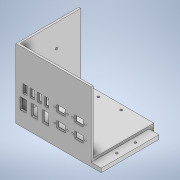
# Autodesk Inventor part: Quarter4
Saved by Autodesk Inventor 2020.2 (Build 242310000, 310)
## iProperties
Created: 2020-01-16
Part Number: Quarter4
Material: Generic
Document SubType Name: Modeling
Designer: ColinP
Density: 1 g/cm^3
Appearance: Default
Author: ColinP
Autodesk Inventor part; units mm, degrees
ref_plane "YZ Plane" through (0, 0, 0) normal (1, 0, 0) x (0, 1, 0)
ref_plane "XZ Plane" through (0, 0, 0) normal (0, 1, 0) x (-1, 0, 0)
ref_plane "XY Plane" through (0, 0, 0) normal (0, 0, 1) x (1, 0, 0)
sketch "Sketch1" plane through (0, 0, 0) normal (0, 1, 0) x (-1, 0, 0)
  line L0 (0, 0) -> (150, 0)
  line L1 (150, 0) -> (150, 125)
  line L2 (150, 125) -> (0, 125)
  line L3 (0, 125) -> (0, 0)
  dimension "d0" = 150
  dimension "d1" = 125
  constraints: 8 end point, 2 parallel, 1 horizontal, 1 perpendicular
  measures "d0" distance of L2.end L1.end
  measures "d1" distance of L1.end L0.end
extrude "Extrusion1" add sketch "Sketch1" along normal blind 10
sketch "Sketch2" plane through (0, 10, 0) normal (0, 1, 0) x (1, 0, 0)
  line L0 (0, -125) -> (0, 0) projected
  line L1 (0, 0) -> (-146, 0)
  line L2 (-146, 0) -> (-146, -121)
  line L3 (-146, -121) -> (0, -121)
  line L4 (0, -121) -> (0, 0)
  line L5 (0, -125) -> (0, 0) projected
  line L6 (0, 0) -> (-150, 0) projected
  line L7 (-150, 0) -> (-150, -125) projected
  line L8 (-150, -125) -> (0, -125) projected
  point P0 (-146, 0)
  dimension "d4" = 146
  dimension "d5" = 121
  constraints: 8 end point, 2 parallel, 1 horizontal, 1 perpendicular
  measures "d4" distance of L3.end L2.end
  measures "d5" distance of L2.end L1.end
extrude "Extrusion2" add sketch "Sketch2" along normal blind 125 contours L8 L7 L6 L2 L3 L0
sketch "Sketch3" plane through (0, 0, 125) normal (1, 0, 0) x (0, 0, -1)
  line L0 (0, 0) -> (0, 135) projected
  line L1 (0, 0) -> (0, 5)
  line L2 (125, 0) -> (125, 10) projected
  line L3 (125, 0) -> (0, 0) projected
  line L4 (125, 0) -> (0, 0)
  line L5 (0, 5) -> (115, 5)
  line L6 (115, 5) -> (125, 5)
  line L7 (115, 5) -> (115, 0)
  line L8 (0, 0) -> (125, 0) projected
  dimension "d8" = 5
  dimension "d95" = 125
  dimension "d96" = 115
  constraints: 10 end point, 2 horizontal, 2 point on line, 1 midpoint, 1 perpendicular
  measures "d8" distance of L0.start L1.end
  measures "d95" distance of L2.start L0.start
  measures "d96" distance of L1.end L5.end
sketch "Sketch4" plane through (0, 10, 121) normal (0, 0, -1) x (-1, 0, 0)
  line L0 (0, 20) -> (16, 20)
  line L1 (16, 20) -> (32.7, 20)
  line L2 (32.7, 20) -> (32.7, 32.9)
  line L3 (32.7, 32.9) -> (16, 32.9)
  line L4 (16, 32.9) -> (16, 20)
  line L5 (16, 26.45) -> (13, 26.45)
  line L6 (13, 26.45) -> (11.5, 26.45)
  circle A0 centre (11.5, 26.45) radius 1.5
  line L7 (32.7, 26.45) -> (37.2, 26.45)
  circle A1 centre (37.2, 26.45) radius 1.5
  line L8 (16, 32.9) -> (16, 47.9)
  line L9 (16, 47.9) -> (32.7, 47.9)
  line L10 (32.7, 47.9) -> (32.7, 60.8)
  line L11 (32.7, 60.8) -> (16, 60.8)
  line L12 (16, 60.8) -> (16, 47.9)
  line L13 (16, 54.35) -> (11.5, 54.35)
  line L14 (11.5, 54.35) -> (37.2, 54.35)
  circle A2 centre (11.5, 54.35) radius 1.5
  circle A3 centre (37.2, 54.35) radius 1.5
  line L15 (47.2, 54.35) -> (51.7, 54.35)
  line L16 (51.7, 54.35) -> (51.7, 47.9)
  line L17 (51.7, 47.9) -> (68.4, 47.9)
  line L18 (68.4, 47.9) -> (68.4, 60.8)
  line L19 (68.4, 60.8) -> (51.7, 60.8)
  line L20 (51.7, 60.8) -> (51.7, 54.35)
  line L21 (68.4, 54.35) -> (72.9, 54.35)
  circle A4 centre (47.2, 54.35) radius 1.5
  circle A5 centre (72.9, 54.35) radius 1.5
  line L22 (0, 0) -> (0, 125) projected
  line L23 (0, 20) -> (0, 0)
  line L24 (51.7, 32.9) -> (51.7, 20)
  line L25 (51.7, 20) -> (68.4, 20)
  line L26 (68.4, 20) -> (68.4, 32.9)
  line L27 (68.4, 32.9) -> (51.7, 32.9)
  line L28 (68.4, 26.45) -> (72.9, 26.45)
  line L29 (72.9, 26.45) -> (47.2, 26.45)
  circle A6 centre (47.2, 26.45) radius 1.5
  circle A7 centre (72.9, 26.45) radius 1.5
  line L30 (68.4, 47.9) -> (68.4, 32.9)
  line L31 (37.2, 54.35) -> (47.2, 54.35)
  point P0 (0, -10)
  dimension "d12" = 16
  dimension "d13" = 16.7
  dimension "d14" = 12.9
  dimension "d15" = 3
  dimension "d16" = 1.5
  dimension "d17" = 4.5
  dimension "d18" = 3
  dimension "d19" = 15
  dimension "d20" = 12.9
  dimension "d23" = 4.5
  dimension "d25" = 4.5
  dimension "d29" = 3
  dimension "d30" = 3
  dimension "d57" = 20
  dimension "d58" = 3
  dimension "d59" = 3
  dimension "d60" = 16.7
  dimension "d62" = 15
  dimension "d73" = 3
  dimension "d74" = 10
  dimension "d75" = 4.5
  dimension "d76" = 16.7
  dimension "d77" = 16.7
  constraints: 62 end point, 17 perpendicular, 8 coincident, 7 centre point, 7 horizontal, 6 point on line, 5 midpoint, 2 collinear, 1 horizontal alignment, 1 vertical, 2 other
  measures "d12" distance of L0.start L0.end
  measures "d13" distance of L0.end L1.end
  measures "d14" distance of L1.end L2.end
  measures "d15" distance of L5.start L5.end
  measures "d16" distance of L5.end L6.end
  measures "d17" distance of L7.start L7.end
  measures "d18" diameter of A1
  measures "d19" distance of L3.end L8.end
  measures "d20" distance of L9.end L10.end
  measures "d23" distance of L15.start L15.end
  measures "d25" distance of L21.start L21.end
  measures "d29" diameter of A4
  measures "d30" diameter of A5
  measures "d57" distance of L0.start L22.start
  measures "d58" diameter of A6
  measures "d59" diameter of A7
  measures "d60" distance of L10.end L11.end
  measures "d62" distance of L17.end L26.end
  measures "d73" diameter of A3
  measures "d74" distance of L31.start L31.end
  measures "d75" distance from line of L10 L14.end
  measures "d76" distance of L26.end L24.start
  measures "d77" distance of L16.end L17.end
extrude "Extrusion4" cut sketch "Sketch4" against normal blind 125 contours L4 L3 L2 L1 | L26 L29 L24 L27 | L20 L19 L18 L17 L16 | L12 L14 L10 L9 | L12 L11 L10 L14 | L26 L25 L24 L29
hole "Hole1" at (-11.5, 64.35, 121) at (-37.2, 64.35, 121) at (-47.2, 64.35, 121) at (-72.9, 64.35, 121) at (-37.2, 36.45, 121) at (-11.5, 36.45, 121) at (-47.2, 36.45, 121) at (-72.9, 36.45, 121) direction (0, 0, 1) diameter 3 end through all
sketch "Sketch5" plane through (-150, 135, 125) normal (0, 0, 1) x (1, 0, 0)
  circle A0 centre (77.1, -70.65) radius 1.5 projected
  line L0 (77.1, -70.65) -> (65.6, -70.65)
  line L1 (65.6, -70.65) -> (65.6, -62.3)
  line L2 (65.6, -62.3) -> (65.6, -79)
  line L3 (65.6, -79) -> (57.5, -79)
  line L4 (57.5, -79) -> (57.5, -62.3)
  line L5 (57.5, -62.3) -> (65.6, -62.3)
  line L6 (57.5, -62.3) -> (51.1, -62.3)
  line L7 (51.1, -62.3) -> (36.6, -62.3)
  line L8 (51.1, -62.3) -> (43, -62.3)
  line L9 (43, -62.3) -> (43, -79)
  line L10 (43, -79) -> (51.1, -79)
  line L11 (51.1, -79) -> (51.1, -62.3)
  line L12 (36.6, -62.3) -> (28.5, -62.3)
  line L13 (28.5, -62.3) -> (28.5, -79)
  line L14 (28.5, -79) -> (36.6, -79)
  line L15 (36.6, -79) -> (36.6, -62.3)
  line L16 (28.5, -62.3) -> (22.1, -62.3)
  line L17 (22.1, -62.3) -> (14, -62.3)
  line L18 (14, -62.3) -> (14, -79)
  line L19 (14, -79) -> (22.1, -79)
  line L20 (22.1, -79) -> (22.1, -62.3)
  point P0 (150, -135)
  point P1 (43, -62.3)
  dimension "d41" = 11.5
  dimension "d43" = 8.35
  dimension "d44" = 16.7
  dimension "d45" = 8.1
  dimension "d46" = 6.4
  dimension "d47" = 14.5
  dimension "d48" = 8.1
  dimension "d49" = 16.7
  dimension "d50" = 8.1
  dimension "d51" = 16.7
  dimension "d52" = 6.4
  dimension "d53" = 8.1
  dimension "d54" = 16.7
  constraints: 42 end point, 6 horizontal, 6 parallel, 6 perpendicular, 2 point on line, 1 vertical
  measures "d41" distance of L0.start L0.end
  measures "d43" distance of L0.end L1.end
  measures "d44" distance of L1.end L2.end
  measures "d45" distance of L2.end L3.end
  measures "d46" distance of L4.end L6.end
  measures "d47" distance of L6.end L7.end
  measures "d48" distance of L10.end L9.end
  measures "d49" distance of L9.end L8.end
  measures "d50" distance of L14.end L13.end
  measures "d51" distance of L13.end L12.end
  measures "d52" distance of L12.end L16.end
  measures "d53" distance of L19.end L18.end
  measures "d54" distance of L18.end L17.end
extrude "Extrusion5" cut sketch "Sketch5" against normal blind 10 contours L20 L19 L18 L17 | L15 L14 L13 L12 | L11 L10 L9 L7 | L2 L3 L4 L5 L1
sketch "Sketch8" plane through (-150, 135, 125) normal (0, 0, 1) x (1, 0, 0)
  circle A0 centre (77.1, -98.55) radius 1.5 projected
  line L0 (77.1, -98.55) -> (65.6, -98.55)
  line L1 (65.6, -98.55) -> (65.6, -87.25)
  line L2 (65.6, -87.25) -> (65.6, -109.85)
  line L3 (65.6, -109.85) -> (53.1, -109.85)
  line L4 (53.1, -109.85) -> (53.1, -87.25)
  line L5 (53.1, -87.25) -> (65.6, -87.25)
  line L6 (53.1, -87.25) -> (43.1, -87.25)
  line L7 (43.1, -87.25) -> (43.1, -109.85)
  line L8 (43.1, -109.85) -> (30.6, -109.85)
  line L9 (30.6, -109.85) -> (30.6, -87.25)
  line L10 (30.6, -87.25) -> (43.1, -87.25)
  line L11 (30.6, -87.25) -> (20.6, -87.25)
  line L12 (20.6, -87.25) -> (20.6, -109.85)
  line L13 (20.6, -109.85) -> (8.1, -109.85)
  line L14 (8.1, -109.85) -> (8.1, -87.25)
  line L15 (8.1, -87.25) -> (20.6, -87.25)
  dimension "d63" = 11.5
  dimension "d64" = 11.3
  dimension "d65" = 22.6
  dimension "d66" = 12.5
  dimension "d67" = 10
  dimension "d68" = 12.5
  dimension "d69" = 10
  dimension "d70" = 22.6
  dimension "d71" = 12.5
  dimension "d113" = 22.6
  constraints: 32 end point, 10 perpendicular, 6 point on line, 2 horizontal
  measures "d63" distance of L0.start L0.end
  measures "d64" distance of L0.end L1.end
  measures "d65" distance of L1.end L2.end
  measures "d66" distance of L2.end L3.end
  measures "d67" distance of L4.end L6.end
  measures "d68" distance of L7.end L8.end
  measures "d69" distance of L9.end L11.end
  measures "d70" distance of L11.end L12.end
  measures "d71" distance of L12.end L13.end
  measures "d113" distance of L13.end L14.end
extrude "Extrusion6" cut sketch "Sketch8" against normal blind 10 contours L12 L13 L14 L15 | L7 L8 L9 L10 | L2 L3 L4 L5 L1
sketch "Sketch9" plane through (-146, 10, 121) normal (1, 0, 0) x (0, 0, -1)
  line L0 (0, 0) -> (0, 125) projected
  line L1 (0, 125) -> (50, 125)
  line L2 (0, 125) -> (121, 125) projected
  line L3 (50, 125) -> (50, 85)
  line L4 (50, 85) -> (95, 85)
  line L5 (95, 85) -> (95, 28)
  line L6 (95, 28) -> (50, 28)
  line L7 (50, 28) -> (50, 85)
  line L8 (72.5, 85) -> (72.5, 80)
  line L9 (72.5, 80) -> (72.5, 33)
  circle A0 centre (72.5, 80) radius 2.5
  circle A1 centre (72.5, 33) radius 2.5
  point P0 (121, -10)
  dimension "d80" = 50
  dimension "d81" = 40
  dimension "d82" = 45
  dimension "d83" = 57
  dimension "d84" = 5
  dimension "d85" = 47
  dimension "d86" = 5
  dimension "d87" = 5
  constraints: 16 end point, 4 perpendicular, 2 centre point, 2 coincident, 2 point on line, 1 horizontal, 1 midpoint, 1 vertical
  measures "d80" distance of L0.end L1.end
  measures "d81" distance of L1.end L3.end
  measures "d82" distance of L3.end L4.end
  measures "d83" distance of L4.end L5.end
  measures "d84" distance of L8.start L8.end
  measures "d85" distance of L8.end L9.end
  measures "d86" diameter of A0
  measures "d87" diameter of A1
hole "Hole2" at (-146, 90, 48.5) at (-146, 43, 48.5) direction (-1, 0, 0) diameter 4.318 end through all
extrude "Extrusion7" add sketch "Sketch3" along normal blind 20 contours L0 L5 L7 L3
sketch "Sketch10" plane through (0, 0, 0) normal (0, -1, 0) x (1, 0, 0)
  point P0 (0, 0)
sketch "Sketch11" plane through (0, 0, 0) normal (0, 0, -1) x (-1, 0, 0)
  line L0 (150, 0) -> (150, 135) projected
  line L1 (150, 0) -> (150, 5)
  line L2 (150, 5) -> (10, 5)
  line L3 (10, 5) -> (10, 0)
  line L4 (10, 0) -> (150, 0)
  point P0 (0, 0)
  dimension "d99" = 5
  dimension "d100" = 140
  constraints: 8 end point, 3 perpendicular, 1 point on line
  measures "d99" distance of L0.start L1.end
  measures "d100" distance of L1.end L2.end
extrude "Extrusion8" cut sketch "Sketch11" against normal blind 20
sketch "Sketch13" plane through (0, 10, 0) normal (0, 1, 0) x (1, 0, 0)
  line L0 (0, 0) -> (-146, 0) projected
  line L1 (0, 0) -> (-10, 0)
  line L2 (-10, 0) -> (-55.3333, 0)
  line L3 (-55.3333, 0) -> (-100.6667, 0)
  line L4 (-100.6667, 0) -> (-100.6667, -10)
  line L5 (-55.3333, 0) -> (-55.3333, -10)
  dimension "d114" = 10
  dimension "d115" = 45.3333
  dimension "d116" = 45.3333
  dimension "d117" = 10
  dimension "d118" = 10
  constraints: 10 end point, 3 point on line, 1 perpendicular, 1 vertical
  measures "d114" distance of L0.start L1.end
  measures "d115" distance of L1.end L2.end
  measures "d116" distance of L2.end L3.end
  measures "d117" distance of L3.end L4.end
  measures "d118" distance of L2.end L5.end
hole "Hole4" at (-100.6667, 10, 10) at (-55.3333, 10, 10) direction (0, -1, 0) diameter 4.318 end through all
sketch "Sketch12" plane through (0, 0, 0) normal (0, 1, 0) x (1, 0, 0)
  line L0 (-146, -121) -> (-146, 0) projected
  line L1 (-146, 0) -> (-106, 0)
  line L2 (0, 0) -> (-146, 0) projected
  line L3 (-106, 0) -> (-106, -70)
  line L4 (-106, -70) -> (-66, -70)
  dimension "d103" = 40
  dimension "d104" = 70
  dimension "d105" = 40
  constraints: 6 end point, 2 perpendicular, 1 point on line
  measures "d103" distance of L0.end L1.end
  measures "d104" distance of L1.end L3.end
  measures "d105" distance of L3.end L4.end
hole "Hole3" at (-66, 0, 70) at (-106, 0, 70) direction (0, 1, 0) diameter 4 end through all counterbore diameter 6 counterbore depth 3
sketch "Sketch16" plane through (0, 0, 0) normal (0, -1, 0) x (1, 0, 0)
  circle A0 centre (-66, 70) radius 3 projected
  circle A1 centre (-106, 70) radius 3 projected
  line L0 (-10, 20) -> (-10, 0) projected
  line L1 (0, 0) -> (-10, 0) projected
  line L2 (0, 10) -> (0, 0) projected
  line L3 (0, 10) -> (20, 10) projected
  line L4 (20, 125) -> (20, 10) projected
  line L5 (-150, 125) -> (20, 125) projected
  line L6 (-150, 20) -> (-150, 125) projected
  line L7 (-150, 20) -> (-10, 20) projected
extrude "Extrusion10" add sketch "Sketch16" along normal blind 3
sketch "Sketch17" plane through (-66, 3, 70) normal (0, -1, 0) x (1, 0, 0)
  circle A0 centre (0, 0) radius 3 projected
  circle A1 centre (0, 0) radius 2 projected
  circle A2 centre (-40, 0) radius 3 projected
  circle A3 centre (-40, 0) radius 2 projected
  point P0 (66, -70)
extrude "Extrusion11" add sketch "Sketch17" along normal blind 3
sketch "Sketch18" plane through (0, -3, 0) normal (0, -1, 0) x (1, 0, 0)
  circle A0 centre (10, 84) radius 1.75 projected
  circle A1 centre (10, 84) radius 1.75
  circle A2 centre (10, 47) radius 1.75 projected
  circle A3 centre (10, 47) radius 1.75
  point P0 (0, 0)
  constraints: 2 centre point, 2 coincident
hole "Hole6" at (10, -3, 47) at (10, -3, 84) direction (0, 1, 0) diameter 4.318 end through all counterbore diameter 7.62 counterbore depth 5.08
body "Solid1"
